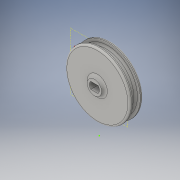
# Autodesk Inventor part: Wheel
Saved by Autodesk Inventor 2016 (Build 200138000, 138)
## iProperties
Created: 2017-09-08
Part Number: Wheel
Material: Generic
Document SubType Name: Modeling
Designer: student
Density: 1 g/cm^3
Appearance: Default
Author: student
Autodesk Inventor part; units mm, degrees
ref_plane "YZ Plane" through (0, 0, 0) normal (1, 0, 0) x (0, 1, 0)
ref_plane "XZ Plane" through (0, 0, 0) normal (0, 1, 0) x (-1, 0, 0)
ref_plane "XY Plane" through (0, 0, 0) normal (0, 0, 1) x (1, 0, 0)
sketch "Sketch8" plane through (0, 0, 0) normal (0, 0, 1) x (1, 0, 0)
  circle A0 centre (0, 0) radius 4.953
  dimension "d46" = 9.906
  constraints: 1 centre point, 1 coincident
  measures "d46" diameter of A0
extrude "Extrusion5" add sketch "Sketch8" along normal blind 2.032
sketch "Sketch9" plane through (0, 0, 0) normal (0, 0, -1) x (-1, 0, 0)
  circle A0 centre (0, 0) radius 22.479
  dimension "d49" = 44.958
  constraints: 1 centre point, 1 coincident
  measures "d49" diameter of A0
extrude "Extrusion6" add sketch "Sketch9" along normal blind 2.032
sketch "Sketch10" plane through (0, 0, -2.032) normal (0, 0, -1) x (-1, 0, 0)
  circle A0 centre (0, 0) radius 19.2405
  dimension "d52" = 38.481
  constraints: 1 centre point, 1 coincident
  measures "d52" diameter of A0
extrude "Extrusion7" add sketch "Sketch10" along normal blind 5.3086
sketch "Sketch11" plane through (0, 0, -7.3406) normal (0, 0, -1) x (-1, 0, 0)
  circle A0 centre (0, 0) radius 22.479
  dimension "d55" = 44.958
  constraints: 1 centre point, 1 coincident
  measures "d55" diameter of A0
extrude "Extrusion8" add sketch "Sketch11" along normal blind 2.032
fillet "Fillet1" radius 1.27 2 edges at (19.2405, 0, -2.032) (19.2405, 0, -7.3406)
sketch "Sketch12" plane through (0, 0, 2.032) normal (0, 0, 1) x (1, 0, 0)
  line L0 (2.5424, 2.413) -> (-2.5424, 2.413)
  line L1 (-2.5424, -2.413) -> (2.5424, -2.413)
  arc A0 (2.5424, -2.413) -> (2.5424, 2.413) centre (0, 0) ccw
  arc A1 (-2.5424, 2.413) -> (-2.5424, -2.413) centre (0, 0) ccw
  constraints: 4 end point, 4 point on circle, 2 centre point, 1 coincident, 1 horizontal, 1 parallel
fillet "Fillet2" radius 2.032 1 edges at (-4.953, 0, 0)
extrude "Extrusion9" cut sketch "Sketch12" against normal blind 5.4864
fillet "Fillet3" radius 1.27 2 edges at (22.479, 0, 0) (22.479, 0, -9.3726)
sketch "Sketch13" plane through (0, 0, -9.3726) normal (0, 0, -1) x (-1, 0, 0)
  line L0 (-11.6631, 16.0922) -> (28.3879, 16.0922) construction
  line L1 (28.3879, 16.0922) -> (28.3879, -23.9394) construction
  line L2 (28.3879, -23.9394) -> (-11.6631, -23.9394) construction
  line L3 (-11.6631, -23.9394) -> (-11.6631, 16.0922) construction
  point P0 (0, 0)
  constraints: 2 other
sketch "Sketch14" plane through (0, 0, -9.3726) normal (0, 0, -1) x (-1, 0, 0)
  arc A0 (2.1554, 2.9693) -> (1.7501, 2.694) centre (2.6554, 1.7971) ccw
  arc A1 (2.1554, 2.9693) -> (2.4765, 3.3822) centre (1.6621, 3.6843) ccw
  arc A2 (2.4765, 3.3822) -> (2.4368, 4.0772) centre (1.6621, 3.6843) ccw
  arc A3 (1.8418, 6.8005) -> (2.4368, 4.0772) centre (13.5072, 7.9224) ccw
  arc A4 (1.7501, 10.1958) -> (1.8418, 6.8005) centre (11.0319, 8.7477) ccw
  arc A5 (2.9104, 12.236) -> (1.7501, 10.1958) centre (6.1526, 9.042) ccw
  arc A6 (6.43, 14.2181) -> (2.9104, 12.236) centre (8.1172, 7.1065) ccw
  arc A7 (10.6207, 14.1034) -> (6.43, 14.2181) centre (8.2042, 2.4297) ccw
  arc A8 (14.0325, 11.983) -> (10.6207, 14.1034) centre (8.6874, 7.1876) ccw
  arc A9 (15.0359, 9.8014) -> (14.0325, 11.983) centre (11.01, 9.2713) ccw
  arc A10 (14.8648, 6.6399) -> (15.0359, 9.8014) centre (-0.413, 9.0519) ccw
  arc A11 (14.2073, 4.0045) -> (14.8648, 6.6399) centre (-0.413, 9.0519) ccw
  arc A12 (14.2073, 4.0045) -> (14.6583, 2.9004) centre (15.1502, 3.7455) ccw
  arc A13 (14.9881, 2.5005) -> (14.6583, 2.9004) centre (14.6531, 2.5602) ccw
  arc A14 (14.245, 0.3081) -> (14.9881, 2.5005) centre (7.393, 3.8527) ccw
  arc A15 (13.7789, 0.0634) -> (14.245, 0.3081) centre (13.7426, 0.6989) ccw
  arc A16 (13.7789, 0.0634) -> (12.303, 0) centre (13.2742, -5.3989) ccw
  arc A17 (12.303, 0) -> (11.5427, -0.2856) centre (12.5075, -1.6994) ccw
  arc A18 (11.5427, -0.2856) -> (11.5009, -0.5189) centre (11.6363, -0.4228) ccw
  arc A19 (11.8518, -0.5637) -> (11.5009, -0.5189) centre (11.5686, -1.3866) ccw
  arc A20 (12.0712, -0.6761) -> (11.8518, -0.5637) centre (11.5686, -1.3866) ccw
  arc A21 (11.7047, -1.7696) -> (12.0712, -0.6761) centre (4.4066, 1.2849) ccw
  arc A22 (10.8127, -2.2848) -> (11.7047, -1.7696) centre (7.6492, 4.2219) ccw
  line L0 (10.8127, -2.2848) -> (10.8127, -1.293)
  line L1 (10.8127, -1.293) -> (10.6646, -1.293)
  line L2 (10.6646, -1.293) -> (10.6646, -2.3547)
  line L3 (10.6646, -2.3547) -> (9.733, -2.7065)
  line L4 (9.733, -2.7065) -> (9.733, -1.5731)
  line L5 (9.733, -1.5731) -> (9.5022, -1.5731)
  line L6 (9.5022, -1.5731) -> (9.5022, -2.819)
  line L7 (9.5022, -2.819) -> (8.4847, -3.1284)
  line L8 (8.4847, -3.1284) -> (8.4847, -1.805)
  line L9 (8.4847, -1.805) -> (8.2367, -1.805)
  line L10 (8.2367, -1.805) -> (8.2367, -3.1284)
  line L11 (8.2367, -3.1284) -> (7.2224, -2.819)
  line L12 (7.2224, -2.819) -> (7.2224, -1.5892)
  line L13 (7.2224, -1.5892) -> (6.9842, -1.5892)
  line L14 (6.9842, -1.5892) -> (6.9842, -2.7463)
  line L15 (6.9842, -2.7463) -> (6.1526, -2.3878)
  line L16 (6.1526, -2.3878) -> (6.0568, -1.293)
  line L17 (6.0568, -1.293) -> (5.9026, -1.293)
  line L18 (5.9026, -1.293) -> (5.9634, -2.2848)
  line L19 (5.9634, -2.2848) -> (5.8672, -2.2848)
  line L20 (5.8672, -2.2848) -> (5.0103, -1.7889)
  line L21 (5.0103, -1.7889) -> (4.6561, -0.6761)
  arc A23 (4.8885, -0.5352) -> (4.6561, -0.6761) centre (4.9286, -0.8633) ccw
  arc A24 (4.8885, -0.5352) -> (5.229, -0.4771) centre (4.851, 0.7128) ccw
  arc A25 (5.229, -0.4771) -> (5.1839, -0.2978) centre (5.1091, -0.412) ccw
  arc A26 (5.1839, -0.2978) -> (4.2016, 0.0442) centre (3.8673, -2.4973) ccw
  arc A27 (4.2016, 0.0442) -> (3.8848, 0.0661) centre (3.8673, -2.4973) ccw
  line L22 (3.8848, 0.0661) -> (2.8994, 0.0661)
  arc A28 (2.458, 0.3081) -> (2.8994, 0.0661) centre (2.9407, 0.6649) ccw
  arc A29 (1.973, 1.6677) -> (2.458, 0.3081) centre (7.1797, 2.759) ccw
  arc A30 (1.7501, 2.3516) -> (1.973, 1.6677) centre (14.1461, 6.0133) ccw
  line L23 (1.7501, 2.3516) -> (1.7501, 2.694)
  line L24 (11.4728, -0.3935) -> (9.3663, 0.3081) construction
  arc A31 (9.3663, 0.3081) -> (9.4802, 0.5895) centre (8.8115, 0.6965) ccw
  arc A32 (9.4802, 0.5895) -> (8.3607, 2.8052) centre (2.0109, -1.7938) ccw
  arc A33 (8.3607, 2.8052) -> (7.2718, 0.7679) centre (16.0314, -2.6042) ccw
  arc A34 (7.2718, 0.7679) -> (7.426, 0.2056) centre (7.8089, 0.6129) ccw
  arc A35 (7.426, 0.2056) -> (7.8856, 0.0816) centre (7.7641, 0.5452) ccw
  arc A36 (8.3607, 0.4651) -> (7.8856, 0.0816) centre (8.5278, -0.228) ccw
  arc A37 (8.8695, 0.0523) -> (8.3607, 0.4651) centre (8.2875, -0.1451) ccw
  arc A38 (8.8695, 0.0523) -> (9.2323, 0.1353) centre (8.9898, 0.3608) ccw
  arc A39 (9.2323, 0.1353) -> (9.3663, 0.3081) centre (8.9522, 0.4907) ccw
  line L25 (2.3047, 3.0998) -> (3.4958, 2.9693) construction
  line L26 (3.4958, 2.9693) -> (3.4958, 4.1245)
  arc A40 (4.2016, 4.7684) -> (3.4958, 4.1245) centre (4.4519, 3.7852) ccw
  arc A41 (5.1839, 4.7684) -> (4.2016, 4.7684) centre (4.6928, 3.3476) ccw
  arc A42 (7.3786, 3.5009) -> (5.1839, 4.7684) centre (2.4987, -2.4152) ccw
  arc A43 (7.2224, 3.2569) -> (7.3786, 3.5009) centre (6.9519, 3.6021) ccw
  arc A44 (5.2415, 2.2282) -> (7.2224, 3.2569) centre (2.8213, 9.3105) ccw
  arc A45 (4.7924, 2.2711) -> (5.2415, 2.2282) centre (5.1511, 3.6558) ccw
  arc A46 (3.4958, 2.9693) -> (4.7924, 2.2711) centre (5.6203, 5.3616) ccw
  arc A47 (9.3938, 3.4781) -> (7.3786, 3.5009) centre (7.9086, -38.7272) ccw construction
  arc A48 (11.9655, 4.8508) -> (9.3938, 3.4781) centre (13.4221, -0.9731) ccw
  arc A49 (13.2527, 4.1814) -> (11.9655, 4.8508) centre (12.1838, 3.6983) ccw
  arc A50 (13.2527, 2.9693) -> (13.2527, 4.1814) centre (5.9292, 3.5753) ccw
  arc A51 (11.9655, 2.2511) -> (13.2527, 2.9693) centre (10.4074, 6.556) ccw
  arc A52 (11.3028, 2.3252) -> (11.9655, 2.2511) centre (11.7552, 3.3707) ccw
  arc A53 (9.995, 2.9288) -> (11.3028, 2.3252) centre (12.8377, 7.3694) ccw
  arc A54 (9.3938, 3.4781) -> (9.995, 2.9288) centre (10.5045, 4.09) ccw
  point P0 (0, 0)
  constraints: 116 point on circle, 55 centre point, 54 end point, 8 perpendicular, 4 concentric, 4 tangent, 3 parallel, 3 vertical, 2 horizontal, 2 point on line
body "Solid2"
